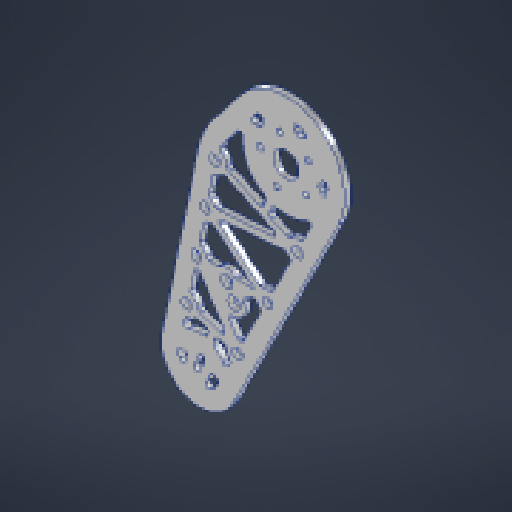
# Autodesk Inventor part: tank_inside_panel
Saved by Autodesk Inventor 2023 (Build 270158000, 158)
## iProperties
Created: 2023-02-28
Part Number: tank_inside_panel
Material: Aluminum 6061
Document SubType Name: Modeling
Designer: ralph
Density: 2.7 g/cm^3
Appearance: Aluminum - Flat
Author: ralph
Autodesk Inventor part; units mm, degrees
(part 1 of 3)
ref_plane "YZ Plane" through (0, 0, 0) normal (1, 0, 0) x (0, 1, 0)
ref_plane "XZ Plane" through (0, 0, 0) normal (0, 1, 0) x (-1, 0, 0)
ref_plane "XY Plane" through (0, 0, 0) normal (0, 0, 1) x (1, 0, 0)
sketch "Sketch1" plane through (0, 0, 0) normal (0, 0, 1) x (1, 0, 0)
  circle A0 centre (-51.8109, -146.0136) radius 3.175 projected
  circle A1 centre (-68.3295, -153.0643) radius 3.175 projected
  line L0 (-87.8947, -227.3231) -> (-92.6287, -239.1078) projected
  arc A2 (-98.521, -236.7409) -> (-92.6287, -239.1078) centre (-95.5749, -237.9244) ccw projected
  line L1 (-98.521, -236.7409) -> (-93.7871, -224.9561) projected
  arc A3 (-87.8947, -227.3231) -> (-93.7871, -224.9561) centre (-90.8409, -226.1396) ccw projected
  circle A4 centre (0, 0) radius 13.4938 projected
  line L2 (-56.4266, -250.7606) -> (56.5866, -28.8133) projected
  arc A5 (56.5866, -28.8133) -> (-50.0843, 39.0361) centre (0, 0) ccw projected
  line L3 (-50.0843, 39.0361) -> (-79.8174, 0.8878) projected
  arc A6 (-79.8174, 0.8878) -> (-94.387, -30.7661) centre (-19.7163, -45.9555) ccw projected
  line L4 (-94.387, -30.7661) -> (-133.6545, -223.8044) projected
  arc A7 (-133.6545, -223.8044) -> (-56.4266, -250.7606) centre (-93.2079, -232.032) ccw projected
  circle A8 centre (-6.7844, 27.1038) radius 3.175 projected
  circle A9 centre (-27.8737, 1.9232) radius 3.175 projected
  circle A10 centre (23.6807, 14.8279) radius 3.175 projected
  circle A11 centre (-10.4425, -25.9152) radius 3.175 projected
  circle A12 centre (21.4199, -17.9397) radius 3.175 projected
  circle A13 centre (12.3652, -76.0452) radius 2.413 projected
  circle A14 centre (-19.9055, -139.4223) radius 2.413 projected
  circle A15 centre (-52.1761, -202.7994) radius 2.413 projected
  line L5 (-60.0746, -215.9418) -> (-61.8773, -219.482) projected
  arc A16 (-67.5567, -219.4404) -> (-61.8773, -219.482) centre (-64.7066, -218.0413) ccw projected
  arc A17 (-109.9237, -202.7115) -> (-105.452, -206.2132) centre (-106.8124, -203.3444) ccw projected
  line L6 (-109.9237, -202.7115) -> (-109.1471, -198.8936) projected
  arc A18 (-106.259, -196.3593) -> (-109.1471, -198.8936) centre (-106.0358, -199.5265) ccw projected
  arc A19 (-106.259, -196.3593) -> (-98.2138, -192.7133) centre (-107.1516, -183.6907) ccw projected
  line L7 (4.4671, -89.1879) -> (-13.923, -125.3043) projected
  arc A20 (-64.7831, -204.3333) -> (-60.7584, -212.1608) centre (-52.1761, -202.7994) ccw projected
  arc A21 (-60.0746, -215.9418) -> (-60.7584, -212.1608) centre (-62.9039, -214.5011) ccw projected
  arc A22 (-92.9229, -119.1359) -> (-91.2544, -122.5971) centre (-89.8116, -119.7688) ccw projected
  line L8 (-92.9229, -119.1359) -> (-88.8946, -99.3326) projected
  arc A23 (-86.0064, -96.7983) -> (-88.8946, -99.3326) centre (-85.7833, -99.9655) ccw projected
  arc A24 (-86.0064, -96.7983) -> (-81.6603, -95.6989) centre (-86.899, -84.1297) ccw projected
  arc A25 (-82.7967, -69.3554) -> (-81.1281, -72.8166) centre (-79.6854, -69.9883) ccw projected
  line L9 (-82.7967, -69.3554) -> (-78.7683, -49.5521) projected
  arc A26 (-75.8802, -47.0178) -> (-78.7683, -49.5521) centre (-75.657, -50.185) ccw projected
  arc A27 (-64.0748, -34.1198) -> (-69.5395, -23.9103) centre (-76.7728, -34.3492) ccw projected
  arc A28 (-70.5556, -19.8503) -> (-69.5395, -23.9103) centre (-67.7312, -21.3006) ccw projected
  arc A29 (-64.7921, -10.8231) -> (-70.5556, -19.8503) centre (-19.7163, -45.9555) ccw projected
  line L10 (-64.7921, -10.8231) -> (-52.5861, 4.8375) projected
  arc A30 (-46.9122, 2.703) -> (-52.5861, 4.8375) centre (-50.0819, 2.8857) ccw projected
  arc A31 (-46.9122, 2.703) -> (-23.4164, -40.7398) centre (0, 0) ccw projected
  arc A32 (26.6735, -45.5766) -> (22.335, -41.3425) centre (23.8442, -44.136) ccw projected
  line L11 (26.6735, -45.5766) -> (18.348, -61.9272) projected
  arc A33 (14.8879, -63.5983) -> (18.348, -61.9272) centre (15.5186, -60.4865) ccw projected
  arc A34 (1.4518, -82.5405) -> (3.7832, -85.4068) centre (12.3652, -76.0452) ccw projected
  arc A35 (4.4671, -89.1879) -> (3.7832, -85.4068) centre (1.6378, -87.7473) ccw projected
  arc A36 (-17.3829, -126.9753) -> (-13.923, -125.3043) centre (-16.7523, -123.8636) ccw projected
  arc A37 (-17.3829, -126.9753) -> (-25.1442, -127.8531) centre (-19.9055, -139.4223) ccw projected
  arc A38 (-63.3886, -164.7638) -> (-63.3439, -164.7448) centre (-68.3295, -153.0643) ccw projected
  line L12 (-63.3439, -164.7448) -> (-46.8252, -157.694) projected
  arc A39 (-46.8252, -157.694) -> (-39.1245, -145.4252) centre (-51.8109, -146.0136) ccw projected
  arc A40 (-35.7266, -142.1112) -> (-39.1245, -145.4252) centre (-35.9529, -145.2781) ccw projected
  line L13 (-35.7266, -142.1112) -> (-34.3965, -142.2063) projected
  arc A41 (-31.6794, -144.183) -> (-34.3965, -142.2063) centre (-34.6229, -145.3732) ccw projected
  arc A42 (-31.6794, -144.183) -> (-28.4876, -148.7838) centre (-19.9055, -139.4223) ccw projected
  arc A43 (-27.8038, -152.5648) -> (-28.4876, -148.7838) centre (-30.6331, -151.1242) ccw projected
  line L14 (-27.8038, -152.5648) -> (-46.1939, -188.6813) projected
  arc A44 (-49.6538, -190.3524) -> (-46.1939, -188.6813) centre (-49.0232, -187.2407) ccw projected
  arc A45 (-49.6538, -190.3524) -> (-50.0192, -190.2839) centre (-52.1761, -202.7994) ccw projected
  arc A46 (-52.1408, -188.8873) -> (-50.0192, -190.2839) centre (-49.48, -187.1551) ccw projected
  line L15 (-52.1408, -188.8873) -> (-64.8141, -169.4209) projected
  arc A47 (-63.3886, -164.7638) -> (-64.8141, -169.4209) centre (-62.1533, -167.6886) ccw projected
  arc A48 (-49.8924, -133.4593) -> (-51.9243, -133.3141) centre (-51.8109, -146.0136) ccw projected
  line L16 (-51.9243, -133.3141) -> (-82.5342, -131.1262) projected
  arc A49 (-85.2514, -129.1495) -> (-82.5342, -131.1262) centre (-82.3079, -127.9593) ccw projected
  arc A50 (-85.2514, -129.1495) -> (-91.2544, -122.5971) centre (-97.0253, -133.9102) ccw projected
  line L17 (-78.3296, -96.1425) -> (-39.1874, -128.4482) projected
  arc A51 (-41.4348, -134.0638) -> (-39.1874, -128.4482) centre (-41.2084, -130.8969) ccw projected
  line L18 (-41.4348, -134.0638) -> (-49.8924, -133.4593) projected
  line L19 (-94.937, -191.9699) -> (-86.0461, -195.0603) projected
  arc A52 (-64.7831, -204.3333) -> (-66.8925, -201.7178) centre (-67.9349, -204.7168) ccw projected
  arc A53 (-94.937, -191.9699) -> (-98.2138, -192.7133) centre (-95.9794, -194.9689) ccw projected
  line L20 (-65.4743, -43.8405) -> (-13.0907, -68.3439) projected
  arc A54 (-14.1782, -74.3844) -> (-13.0907, -68.3439) centre (-14.436, -71.2199) ccw projected
  line L21 (-14.1782, -74.3844) -> (-72.9996, -79.1751) projected
  arc A55 (-75.9857, -77.6344) -> (-72.9996, -79.1751) centre (-73.2574, -76.0105) ccw projected
  arc A56 (-75.9857, -77.6344) -> (-81.1281, -72.8166) centre (-86.899, -84.1297) ccw projected
  arc A57 (-65.4743, -43.8405) -> (-68.8102, -44.243) centre (-66.8195, -46.7164) ccw projected
  line L22 (-28.4749, -127.4095) -> (-71.2037, -92.1436) projected
  arc A58 (-69.4404, -86.5304) -> (-71.2037, -92.1436) centre (-69.1827, -89.6949) ccw projected
  line L23 (-69.4404, -86.5304) -> (-1.5342, -80.9998) projected
  arc A59 (1.4518, -82.5405) -> (-1.5342, -80.9998) centre (-1.2765, -84.1643) ccw projected
  arc A60 (-28.4749, -127.4095) -> (-25.1442, -127.8531) centre (-26.4539, -124.9608) ccw projected
  arc A61 (14.8879, -63.5983) -> (4.4026, -66.1514) centre (12.3652, -76.0452) ccw projected
  arc A62 (1.0667, -66.5539) -> (4.4026, -66.1514) centre (2.4119, -63.6779) ccw projected
  line L24 (1.0667, -66.5539) -> (-16.1603, -58.4956) projected
  arc A63 (-64.0748, -34.1198) -> (-62.2456, -36.9383) centre (-60.9004, -34.0624) ccw projected
  arc A64 (-61.0938, -193.7571) -> (-61.1139, -193.7769) centre (-52.1761, -202.7994) ccw projected
  arc A65 (-64.3907, -194.5202) -> (-61.1139, -193.7769) centre (-63.3483, -191.5212) ccw projected
  line L25 (-64.3907, -194.5202) -> (-92.4352, -184.7723) projected
  arc A66 (-94.5445, -182.1568) -> (-92.4352, -184.7723) centre (-91.3928, -181.7733) ccw projected
  arc A67 (-94.5445, -182.1568) -> (-101.3806, -172.3776) centre (-107.1516, -183.6907) ccw projected
  arc A68 (-103.0492, -168.9165) -> (-101.3806, -172.3776) centre (-99.9379, -169.5493) ccw projected
  line L26 (-103.0492, -168.9165) -> (-99.0208, -149.1131) projected
  arc A69 (-96.1327, -146.5788) -> (-99.0208, -149.1131) centre (-95.9095, -149.746) ccw projected
  arc A70 (-96.1327, -146.5788) -> (-92.3649, -145.7242) centre (-97.0253, -133.9102) ccw projected
  arc A71 (-88.5389, -146.9454) -> (-92.3649, -145.7242) centre (-91.1997, -148.6777) ccw projected
  line L27 (-88.5389, -146.9454) -> (-60.6625, -189.7642) projected
  arc A72 (-61.0938, -193.7571) -> (-60.6625, -189.7642) centre (-63.3233, -191.4965) ccw projected
  arc A73 (-88.6509, -203.8227) -> (-105.452, -206.2132) centre (-93.2079, -232.032) ccw projected
  line L28 (-22.0524, -44.676) -> (-24.5425, -50.8749) projected
  line L29 (-28.8339, -52.5673) -> (-62.2456, -36.9383) projected
  line L30 (-84.1423, -199.2428) -> (-85.1984, -201.8718) projected
  line L31 (-17.7613, -54.4362) -> (-14.9815, -47.5164) projected
  line L32 (-72.8356, -199.6521) -> (-66.8925, -201.7178) projected
  arc A74 (-67.5567, -219.4404) -> (-76.984, -208.5093) centre (-93.2079, -232.032) ccw projected
  arc A75 (-75.8802, -47.0178) -> (-68.8102, -44.243) centre (-76.7728, -34.3492) ccw projected
  line L33 (-78.1275, -204.7122) -> (-76.8242, -201.4676) projected
  arc A76 (-11.2736, -45.6176) -> (22.335, -41.3425) centre (0, 0) ccw projected
  arc A77 (-84.1423, -199.2428) -> (-86.0461, -195.0603) centre (-87.0885, -198.0593) ccw projected
  arc A78 (-88.6509, -203.8227) -> (-85.1984, -201.8718) centre (-88.1445, -200.6883) ccw projected
  arc A79 (-22.0524, -44.676) -> (-23.4164, -40.7398) centre (-24.9986, -43.4925) ccw projected
  arc A80 (-28.8339, -52.5673) -> (-24.5425, -50.8749) centre (-27.4887, -49.6914) ccw projected
  arc A81 (-78.3296, -96.1425) -> (-81.6603, -95.6989) centre (-80.3506, -98.5912) ccw projected
  arc A82 (-72.8356, -199.6521) -> (-76.8242, -201.4676) centre (-73.878, -202.6511) ccw projected
  arc A83 (-78.1275, -204.7122) -> (-76.984, -208.5093) centre (-75.1814, -205.8957) ccw projected
  arc A84 (-11.2736, -45.6176) -> (-14.9815, -47.5164) centre (-12.0354, -48.6999) ccw projected
  arc A85 (-17.7613, -54.4362) -> (-16.1603, -58.4956) centre (-14.8151, -55.6197) ccw projected
  arc A86 (-115.2631, -229.2902) -> (-114.4847, -238.4545) centre (-93.2079, -232.032) ccw projected
  arc A87 (-113.3713, -227.9304) -> (-115.2631, -229.2902) centre (-113.6877, -229.486) ccw projected
  line L34 (-113.3713, -227.9304) -> (-109.5924, -228.6991) projected
  arc A88 (-107.2952, -233.0332) -> (-109.5924, -228.6991) centre (-110.2253, -231.8104) ccw projected
  arc A89 (-107.2952, -233.0332) -> (-108.2711, -237.6145) centre (-95.5749, -237.9244) ccw projected
  arc A90 (-114.4847, -238.4545) -> (-108.2711, -237.6145) centre (-111.4451, -237.537) ccw projected
  arc A91 (-82.9809, -239.5618) -> (-81.2537, -236.3199) centre (-93.2079, -232.032) ccw projected
  arc A92 (-79.039, -235.4413) -> (-81.2537, -236.3199) centre (-79.7594, -236.8559) ccw projected
  line L35 (-79.039, -235.4413) -> (-73.2785, -238.3744) projected
  arc A93 (-72.5842, -240.5094) -> (-73.2785, -238.3744) centre (-73.9989, -239.7891) ccw projected
  line L36 (-72.5842, -240.5094) -> (-73.4026, -242.1166) projected
  arc A94 (-82.2866, -251.3886) -> (-73.4026, -242.1166) centre (-93.2079, -232.032) ccw projected
  arc A95 (-86.1924, -246.4835) -> (-82.2866, -251.3886) centre (-83.8468, -248.6233) ccw projected
  arc A96 (-86.1924, -246.4835) -> (-82.9809, -239.5618) centre (-95.5749, -237.9244) ccw projected
  line L37 (-36.7385, 25.1704) -> (-35.059, 27.3253) projected
  arc A97 (-31.1029, 31.7555) -> (-35.059, 27.3253) centre (0, 0) ccw projected
  arc A98 (-25.7245, 29.1468) -> (-31.1029, 31.7555) centre (-28.8812, 29.4873) ccw projected
  arc A99 (-25.7245, 29.1468) -> (-25.6629, 24.5535) centre (-6.7844, 27.1038) ccw projected
  arc A100 (-28.6757, 20.9563) -> (-25.6629, 24.5535) centre (-28.8093, 24.1285) ccw projected
  arc A101 (-28.6757, 20.9563) -> (-33.3257, 20.1764) centre (-27.8737, 1.9232) ccw projected
  arc A102 (-36.7385, 25.1704) -> (-33.3257, 20.1764) centre (-34.2343, 23.2186) ccw projected
  arc A103 (35.5169, -0.0989) -> (38.7459, 3.1685) centre (23.6807, 14.8279) ccw projected
  arc A104 (44.4304, 1.3195) -> (38.7459, 3.1685) centre (41.2568, 1.2252) ccw projected
  arc A105 (43.8282, -7.409) -> (44.4304, 1.3195) centre (0, 0) ccw projected
  arc A106 (37.9436, -8.4597) -> (43.8282, -7.409) centre (40.6976, -6.8798) ccw projected
  arc A107 (37.9436, -8.4597) -> (35.1939, -4.7799) centre (21.4199, -17.9397) ccw projected
  arc A108 (35.5169, -0.0989) -> (35.1939, -4.7799) centre (37.4896, -2.5866) ccw projected
  arc A109 (11.0693, 33.748) -> (8.9598, 37.8287) centre (-6.7844, 27.1038) ccw projected
  arc A110 (12.4749, 42.6636) -> (8.9598, 37.8287) centre (11.5838, 39.6162) ccw projected
  arc A111 (20.59, 39.3936) -> (12.4749, 42.6636) centre (0, 0) ccw projected
  arc A112 (19.7709, 33.4723) -> (20.59, 39.3936) centre (19.1193, 36.5798) ccw projected
  arc A113 (19.7709, 33.4723) -> (15.4215, 31.9943) centre (23.6807, 14.8279) ccw projected
  arc A114 (11.0693, 33.748) -> (15.4215, 31.9943) centre (14.045, 34.8554) ccw projected
  point P0 (0, 0)
  point P1 (-30.4878, -157.8365)
  point P2 (-86.8989, -84.1298)
  point P3 (-76.7727, -34.3493)
  point P4 (-67.7312, -21.3007)
  point P5 (0, 0)
  constraints: 1 other
extrude "Extrusion1" add sketch "Sketch1" along normal blind 6.35 contours A7 L4 A6 L3 A5 L2 | A8 | A9 | A10 | A11 | A12 | A13 | A14 | A15 | L5 A16 A74 A83 L33 A82 L32 A52 A20 A21 | L6 A18 A19 A53 L19 A77 L30 A78 A73 A17 | L7 A36 A37 A60 L22 A58 L23 A59 A34 A35 | L8 A23 A24 A81 L17 A51 L18 A48 L16 A49 A50 A22 | L9 A26 A75 A57 L20 A54 L21 A55 A56 A25 | A27 A28 A29 L10 A30 A31 A79 L28 A80 L29 A63 | L11 A33 A61 A62 L24 A85 L31 A84 A76 A32 | A38 L12 A39 A40 L13 A41 A42 A43 L14 A44 A45 A46 L15 A47 | A64 A65 L25 A66 A67 A68 L26 A69 A70 A71 L27 A72 | A87 L34 A88 A89 A90 A86 | A91 A92 L35 A93 L36 A94 A95 A96 | L37 A97 A98 A99 A100 A101 A102 | A103 A104 A105 A106 A107 A108 | A109 A110 A111 A112 A113 A114
sketch "Sketch2" plane through (0, 0, 6.35) normal (0, 0, 1) x (1, 0, 0)
  line L0 (-92.6287, -239.1078) -> (-87.8947, -227.3231) projected
  arc A0 (-87.8947, -227.3231) -> (-93.7871, -224.9561) centre (-90.8409, -226.1396) ccw projected
  line L1 (-93.7871, -224.9561) -> (-98.521, -236.7409) projected
  arc A1 (-98.521, -236.7409) -> (-92.6287, -239.1078) centre (-95.5749, -237.9244) ccw projected
  circle A2 centre (0, 0) radius 13.4938 projected
  line L2 (-56.4266, -250.7606) -> (56.5866, -28.8133) projected
  arc A3 (-133.6545, -223.8044) -> (-56.4266, -250.7606) centre (-93.2079, -232.032) ccw projected
  line L3 (-94.387, -30.7661) -> (-133.6545, -223.8044) projected
  arc A4 (-79.8174, 0.8878) -> (-94.387, -30.7661) centre (-19.7163, -45.9555) ccw projected
  line L4 (-50.0843, 39.0361) -> (-79.8174, 0.8878) projected
  arc A5 (56.5866, -28.8133) -> (-50.0843, 39.0361) centre (0, 0) ccw projected
  circle A6 centre (-10.4425, -25.9152) radius 6.731 projected
  circle A7 centre (-6.7844, 27.1038) radius 6.731 projected
  circle A8 centre (-51.8109, -146.0136) radius 6.731 projected
  circle A9 centre (-68.3295, -153.0643) radius 6.731 projected
  circle A10 centre (23.6807, 14.8279) radius 6.731 projected
  circle A11 centre (-27.8737, 1.9232) radius 6.731 projected
  circle A12 centre (21.4199, -17.9397) radius 6.731 projected
  circle A13 centre (-19.9049, -139.4226) radius 5.588 projected
  circle A14 centre (-52.1756, -202.7997) radius 5.588 projected
  circle A15 centre (12.3657, -76.0454) radius 5.588 projected
  arc A16 (-64.7826, -204.3336) -> (-60.7582, -212.1607) centre (-52.1756, -202.7997) ccw projected
  line L5 (18.3479, -61.9273) -> (26.6735, -45.5766) projected
  arc A17 (-94.5445, -182.1568) -> (-101.3806, -172.3776) centre (-107.1516, -183.6907) ccw projected
  arc A18 (-106.259, -196.3593) -> (-109.1471, -198.8936) centre (-106.0358, -199.5265) ccw projected
  line L6 (-109.1471, -198.8936) -> (-109.9237, -202.7115) projected
  arc A19 (-109.9237, -202.7115) -> (-105.452, -206.2132) centre (-106.8124, -203.3444) ccw projected
  arc A20 (-67.5567, -219.4404) -> (-61.8773, -219.482) centre (-64.7066, -218.0413) ccw projected
  line L7 (-61.8773, -219.482) -> (-60.0745, -215.9416) projected
  arc A21 (-60.0745, -215.9416) -> (-60.7582, -212.1607) centre (-62.9039, -214.5009) ccw projected
  arc A22 (-17.3829, -126.9755) -> (-25.1437, -127.8534) centre (-19.9049, -139.4226) ccw projected
  arc A23 (-17.3829, -126.9755) -> (-13.923, -125.3044) centre (-16.7524, -123.8637) ccw projected
  line L8 (-13.923, -125.3044) -> (4.4672, -89.1877) projected
  arc A24 (4.4672, -89.1877) -> (3.7834, -85.4067) centre (1.6379, -87.7471) ccw projected
  arc A25 (14.888, -63.5984) -> (4.4031, -66.1516) centre (12.3657, -76.0454) ccw projected
  arc A26 (14.888, -63.5984) -> (18.3479, -61.9273) centre (15.5186, -60.4867) ccw projected
  arc A27 (26.6735, -45.5766) -> (22.335, -41.3425) centre (23.8442, -44.136) ccw projected
  arc A28 (-11.2736, -45.6176) -> (22.335, -41.3425) centre (0, 0) ccw projected
  arc A29 (-46.9122, 2.703) -> (-52.5861, 4.8375) centre (-50.0819, 2.8857) ccw projected
  line L9 (-52.5861, 4.8375) -> (-64.7921, -10.8231) projected
  arc A30 (-64.7921, -10.8231) -> (-70.5556, -19.8503) centre (-19.7163, -45.9555) ccw projected
  arc A31 (-70.5556, -19.8503) -> (-69.5395, -23.9103) centre (-67.7312, -21.3006) ccw projected
  arc A32 (-64.0748, -34.1198) -> (-69.5395, -23.9103) centre (-76.7728, -34.3492) ccw projected
  arc A33 (-75.8802, -47.0178) -> (-78.7683, -49.5521) centre (-75.657, -50.185) ccw projected
  line L10 (-78.7683, -49.5521) -> (-82.7967, -69.3554) projected
  arc A34 (-82.7967, -69.3554) -> (-81.1281, -72.8166) centre (-79.6854, -69.9883) ccw projected
  arc A35 (-86.0064, -96.7983) -> (-81.6603, -95.6989) centre (-86.899, -84.1297) ccw projected
  arc A36 (-86.0064, -96.7983) -> (-88.8946, -99.3326) centre (-85.7833, -99.9655) ccw projected
  line L11 (-88.8946, -99.3326) -> (-92.9229, -119.1359) projected
  arc A37 (-92.9229, -119.1359) -> (-91.2544, -122.5971) centre (-89.8116, -119.7688) ccw projected
  line L12 (-60.662, -189.7645) -> (-88.5389, -146.9454) projected
  arc A38 (-88.5389, -146.9454) -> (-92.3648, -145.7242) centre (-91.1997, -148.6777) ccw projected
  arc A39 (-96.1327, -146.5788) -> (-92.3648, -145.7242) centre (-97.0253, -133.9102) ccw projected
  arc A40 (-96.1327, -146.5788) -> (-99.0208, -149.1131) centre (-95.9095, -149.746) ccw projected
  line L13 (-99.0208, -149.1131) -> (-103.0492, -168.9165) projected
  arc A41 (-103.0492, -168.9165) -> (-101.3806, -172.3776) centre (-99.9379, -169.5493) ccw projected
  arc A42 (-94.5445, -182.1568) -> (-92.4352, -184.7724) centre (-91.3928, -181.7734) ccw projected
  line L14 (-92.4352, -184.7724) -> (-64.3901, -194.5205) projected
  arc A43 (-64.3901, -194.5205) -> (-61.1133, -193.7771) centre (-63.3477, -191.5215) ccw projected
  arc A44 (-61.0933, -193.7574) -> (-61.1133, -193.7771) centre (-52.1756, -202.7997) ccw projected
  arc A45 (-61.0933, -193.7574) -> (-60.662, -189.7645) centre (-63.3228, -191.4968) ccw projected
  line L15 (-39.187, -128.4483) -> (-78.3296, -96.1425) projected
  arc A46 (-85.2514, -129.1495) -> (-91.2544, -122.5971) centre (-97.0253, -133.9102) ccw projected
  arc A47 (-85.2514, -129.1495) -> (-82.5342, -131.1263) centre (-82.3079, -127.9594) ccw projected
  line L16 (-82.5342, -131.1263) -> (-51.9258, -133.3141) projected
  arc A48 (-49.8908, -133.4595) -> (-51.9258, -133.3141) centre (-51.8109, -146.0136) ccw projected
  line L17 (-49.8908, -133.4595) -> (-41.4344, -134.064) projected
  arc A49 (-41.4344, -134.064) -> (-39.187, -128.4483) centre (-41.208, -130.8971) ccw projected
  line L18 (-34.396, -142.2065) -> (-35.7265, -142.1114) projected
  arc A50 (-35.7265, -142.1114) -> (-39.1245, -145.4254) centre (-35.9529, -145.2783) ccw projected
  arc A51 (-46.8252, -157.694) -> (-39.1245, -145.4254) centre (-51.8109, -146.0136) ccw projected
  line L19 (-46.8252, -157.694) -> (-63.3439, -164.7448) projected
  arc A52 (-63.3884, -164.7637) -> (-63.3439, -164.7448) centre (-68.3295, -153.0643) ccw projected
  arc A53 (-63.3884, -164.7637) -> (-64.8139, -169.4208) centre (-62.1531, -167.6885) ccw projected
  line L20 (-64.8139, -169.4208) -> (-52.1403, -188.8876) projected
  arc A54 (-52.1403, -188.8876) -> (-50.0187, -190.2842) centre (-49.4795, -187.1553) ccw projected
  arc A55 (-49.6537, -190.3526) -> (-50.0187, -190.2842) centre (-52.1756, -202.7997) ccw projected
  arc A56 (-49.6537, -190.3526) -> (-46.194, -188.6815) centre (-49.0233, -187.2408) ccw projected
  line L21 (-46.194, -188.6815) -> (-27.8037, -152.5647) projected
  arc A57 (-27.8037, -152.5647) -> (-28.4874, -148.7837) centre (-30.633, -151.124) ccw projected
  arc A58 (-31.6789, -144.1832) -> (-28.4874, -148.7837) centre (-19.9049, -139.4226) ccw projected
  arc A59 (-31.6789, -144.1832) -> (-34.396, -142.2065) centre (-34.6224, -145.3734) ccw projected
  arc A60 (-106.259, -196.3593) -> (-98.2138, -192.7133) centre (-107.1516, -183.6907) ccw projected
  arc A61 (-64.7826, -204.3336) -> (-66.8919, -201.7181) centre (-67.9343, -204.7171) ccw projected
  line L22 (-86.0461, -195.0603) -> (-94.937, -191.97) projected
  arc A62 (-94.937, -191.97) -> (-98.2138, -192.7133) centre (-95.9794, -194.969) ccw projected
  line L23 (-16.1603, -58.4956) -> (1.0672, -66.5541) projected
  arc A63 (1.0672, -66.5541) -> (4.4031, -66.1516) centre (2.4125, -63.6782) ccw projected
  arc A64 (-64.0748, -34.1198) -> (-62.2456, -36.9383) centre (-60.9004, -34.0624) ccw projected
  arc A65 (-75.8802, -47.0178) -> (-68.8102, -44.243) centre (-76.7728, -34.3492) ccw projected
  arc A66 (-75.9857, -77.6344) -> (-81.1281, -72.8166) centre (-86.899, -84.1297) ccw projected
  arc A67 (-75.9857, -77.6344) -> (-72.9996, -79.1751) centre (-73.2574, -76.0106) ccw projected
  line L24 (-72.9996, -79.1751) -> (-14.1778, -74.3846) projected
  arc A68 (-14.1778, -74.3846) -> (-13.0903, -68.3441) centre (-14.4355, -71.22) ccw projected
  line L25 (-13.0903, -68.3441) -> (-65.4743, -43.8405) projected
  arc A69 (-65.4743, -43.8405) -> (-68.8102, -44.243) centre (-66.8195, -46.7164) ccw projected
  arc A70 (1.4524, -82.5407) -> (3.7834, -85.4067) centre (12.3657, -76.0454) ccw projected
  arc A71 (1.4524, -82.5407) -> (-1.5337, -81) centre (-1.276, -84.1646) ccw projected
  line L26 (-1.5337, -81) -> (-69.4403, -86.5305) projected
  arc A72 (-69.4403, -86.5305) -> (-71.2036, -92.1437) centre (-69.1826, -89.695) ccw projected
  line L27 (-71.2036, -92.1437) -> (-28.4744, -127.4098) projected
  arc A73 (-28.4744, -127.4098) -> (-25.1437, -127.8534) centre (-26.4534, -124.9611) ccw projected
  arc A74 (-67.5567, -219.4404) -> (-76.984, -208.5093) centre (-93.2079, -232.032) ccw projected
  line L28 (-66.8919, -201.7181) -> (-72.8356, -199.6521) projected
  line L29 (-14.9815, -47.5164) -> (-17.7613, -54.4362) projected
  line L30 (-76.8242, -201.4676) -> (-78.1275, -204.7122) projected
  line L31 (-24.5425, -50.8749) -> (-22.0524, -44.676) projected
  arc A75 (-88.6509, -203.8227) -> (-105.452, -206.2132) centre (-93.2079, -232.032) ccw projected
  line L32 (-85.1984, -201.8718) -> (-84.1423, -199.2428) projected
  arc A76 (-46.9122, 2.703) -> (-23.4164, -40.7398) centre (0, 0) ccw projected
  line L33 (-62.2456, -36.9383) -> (-28.8339, -52.5673) projected
  arc A77 (-72.8356, -199.6521) -> (-76.8242, -201.4676) centre (-73.878, -202.6511) ccw projected
  arc A78 (-78.1275, -204.7122) -> (-76.984, -208.5093) centre (-75.1814, -205.8957) ccw projected
  arc A79 (-11.2736, -45.6176) -> (-14.9815, -47.5164) centre (-12.0354, -48.6999) ccw projected
  arc A80 (-17.7613, -54.4362) -> (-16.1603, -58.4956) centre (-14.8151, -55.6197) ccw projected
  arc A81 (-78.3296, -96.1425) -> (-81.6603, -95.6989) centre (-80.3506, -98.5912) ccw projected
  arc A82 (-84.1423, -199.2428) -> (-86.0461, -195.0603) centre (-87.0885, -198.0593) ccw projected
  arc A83 (-88.6509, -203.8227) -> (-85.1984, -201.8718) centre (-88.1445, -200.6883) ccw projected
  arc A84 (-22.0524, -44.676) -> (-23.4164, -40.7398) centre (-24.9986, -43.4925) ccw projected
  arc A85 (-28.8339, -52.5673) -> (-24.5425, -50.8749) centre (-27.4887, -49.6914) ccw projected
  arc A86 (-82.2866, -251.3886) -> (-73.4026, -242.1166) centre (-93.2079, -232.032) ccw projected
  line L34 (-73.4026, -242.1166) -> (-72.5842, -240.5094) projected
  arc A87 (-72.5842, -240.5094) -> (-73.2785, -238.3744) centre (-73.9989, -239.7891) ccw projected
  line L35 (-73.2785, -238.3744) -> (-79.039, -235.4413) projected
  arc A88 (-79.039, -235.4413) -> (-81.2537, -236.3199) centre (-79.7594, -236.8559) ccw projected
  arc A89 (-82.9809, -239.5618) -> (-81.2537, -236.3199) centre (-93.2079, -232.032) ccw projected
  arc A90 (-86.1924, -246.4835) -> (-82.9809, -239.5618) centre (-95.5749, -237.9244) ccw projected
  arc A91 (-86.1924, -246.4835) -> (-82.2866, -251.3886) centre (-83.8468, -248.6233) ccw projected
  arc A92 (-107.2952, -233.0332) -> (-109.5924, -228.6991) centre (-110.2253, -231.8104) ccw projected
  line L36 (-109.5924, -228.6991) -> (-113.3713, -227.9304) projected
  arc A93 (-113.3713, -227.9304) -> (-115.2631, -229.2902) centre (-113.6877, -229.486) ccw projected
  arc A94 (-115.2631, -229.2902) -> (-114.4847, -238.4545) centre (-93.2079, -232.032) ccw projected
  arc A95 (-114.4847, -238.4545) -> (-108.2711, -237.6145) centre (-111.4451, -237.537) ccw projected
  arc A96 (-107.2952, -233.0332) -> (-108.2711, -237.6145) centre (-95.5749, -237.9244) ccw projected
  arc A97 (35.5169, -0.0989) -> (38.7459, 3.1685) centre (23.6807, 14.8279) ccw projected
  arc A98 (35.5169, -0.0989) -> (35.1939, -4.7799) centre (37.4896, -2.5866) ccw projected
  arc A99 (37.9436, -8.4597) -> (35.1939, -4.7799) centre (21.4199, -17.9397) ccw projected
  arc A100 (37.9436, -8.4597) -> (43.8282, -7.409) centre (40.6976, -6.8798) ccw projected
  arc A101 (43.8282, -7.409) -> (44.4304, 1.3195) centre (0, 0) ccw projected
  arc A102 (44.4304, 1.3195) -> (38.7459, 3.1685) centre (41.2568, 1.2252) ccw projected
  arc A103 (11.0693, 33.748) -> (8.9598, 37.8287) centre (-6.7844, 27.1038) ccw projected
  arc A104 (11.0693, 33.748) -> (15.4215, 31.9943) centre (14.045, 34.8554) ccw projected
  arc A105 (19.7709, 33.4723) -> (15.4215, 31.9943) centre (23.6807, 14.8279) ccw projected
  arc A106 (19.7709, 33.4723) -> (20.59, 39.3936) centre (19.1193, 36.5798) ccw projected
  arc A107 (20.59, 39.3936) -> (12.4749, 42.6636) centre (0, 0) ccw projected
  arc A108 (12.4749, 42.6636) -> (8.9598, 37.8287) centre (11.5838, 39.6162) ccw projected
  arc A109 (-31.1029, 31.7555) -> (-35.059, 27.3253) centre (0, 0) ccw projected
  line L37 (-35.059, 27.3253) -> (-36.7385, 25.1704) projected
  arc A110 (-36.7385, 25.1704) -> (-33.3257, 20.1764) centre (-34.2343, 23.2186) ccw projected
  arc A111 (-28.6757, 20.9563) -> (-33.3257, 20.1764) centre (-27.8737, 1.9232) ccw projected
  arc A112 (-28.6757, 20.9563) -> (-25.6629, 24.5535) centre (-28.8093, 24.1285) ccw projected
  arc A113 (-25.7245, 29.1468) -> (-25.6629, 24.5535) centre (-6.7844, 27.1038) ccw projected
  arc A114 (-25.7245, 29.1468) -> (-31.1029, 31.7555) centre (-28.8812, 29.4873) ccw projected
  point P0 (0, 0)
  point P1 (-30.4878, -157.8365)
  point P2 (-86.8983, -84.1302)
  point P3 (0.0004, -0.0002)
extrude "Extrusion2" [suppressed]
sketch "Sketch3" plane through (0, 0, 6.35) normal (0, 0, 1) x (1, 0, 0)
  arc A0 (56.5866, -28.8133) -> (-50.0843, 39.0361) centre (0, 0) ccw projected
  line L0 (-50.0843, 39.0361) -> (-79.8174, 0.8878) projected
  arc A1 (-79.8174, 0.8878) -> (-94.387, -30.7661) centre (-19.7163, -45.9555) ccw projected
  line L1 (-94.387, -30.7661) -> (-133.6545, -223.8044) projected
  arc A2 (-133.6545, -223.8044) -> (-56.4266, -250.7606) centre (-93.2079, -232.032) ccw projected
  line L2 (-56.4266, -250.7606) -> (56.5866, -28.8133) projected
  circle A3 centre (-51.8109, -146.0136) radius 3.175 projected
  circle A4 centre (-68.3295, -153.0643) radius 3.175 projected
  circle A5 centre (0, 0) radius 13.4938 projected
  line L3 (-98.521, -236.7409) -> (-93.7871, -224.9561) projected
  arc A6 (-87.8947, -227.3231) -> (-93.7871, -224.9561) centre (-90.8409, -226.1396) ccw projected
  line L4 (-87.8947, -227.3231) -> (-92.6287, -239.1078) projected
  arc A7 (-98.521, -236.7409) -> (-92.6287, -239.1078) centre (-95.5749, -237.9244) ccw projected
  circle A8 centre (-51.8109, -146.0136) radius 3.175 projected
  line L5 (-51.8109, -146.0136) -> (-63.5956, -141.2796)
  line L6 (-63.5956, -141.2796) -> (-68.3295, -153.0643)
  line L7 (-51.8109, -146.0136) -> (-56.5448, -157.7983)
  line L8 (-56.5448, -157.7983) -> (-68.3295, -153.0643)
  circle A9 centre (-56.5448, -157.7983) radius 3.175
  circle A10 centre (-63.5956, -141.2796) radius 3.175
  point P0 (0, 0)
  dimension "d4" = 6.35
  dimension "d5" = 6.35
  constraints: 8 end point, 4 perpendicular, 2 centre point, 2 coincident
  measures "d4" diameter of A9
  measures "d5" diameter of A10
extrude "Extrusion3" cut sketch "Sketch3" against normal blind 6.35 contours A10 L6 L5 | L5 L6 A10 | A9 L8 L7 | L7 L8 A9
sketch "Sketch4" plane through (0, 0, 6.35) normal (0, 0, 1) x (1, 0, 0)
  circle A0 centre (-56.5448, -157.7983) radius 3.175 projected
  circle A1 centre (-63.5956, -141.2796) radius 3.175 projected
  arc A2 (56.5866, -28.8133) -> (-50.0843, 39.0361) centre (0, 0) ccw projected
  line L0 (-50.0843, 39.0361) -> (-79.8174, 0.8878) projected
  arc A3 (-79.8174, 0.8878) -> (-94.387, -30.7661) centre (-19.7163, -45.9555) ccw projected
  line L1 (-94.387, -30.7661) -> (-133.6545, -223.8044) projected
  arc A4 (-133.6545, -223.8044) -> (-56.4266, -250.7606) centre (-93.2079, -232.032) ccw projected
  line L2 (-56.4266, -250.7606) -> (56.5866, -28.8133) projected
  circle A5 centre (-51.8109, -146.0136) radius 3.175 projected
  circle A6 centre (-68.3295, -153.0643) radius 3.175 projected
  circle A7 centre (0, 0) radius 13.4938 projected
  line L3 (-98.521, -236.7409) -> (-93.7871, -224.9561) projected
  arc A8 (-87.8947, -227.3231) -> (-93.7871, -224.9561) centre (-90.8409, -226.1396) ccw projected
  line L4 (-87.8947, -227.3231) -> (-92.6287, -239.1078) projected
  arc A9 (-98.521, -236.7409) -> (-92.6287, -239.1078) centre (-95.5749, -237.9244) ccw projected
  point P0 (0, 0)
extrude "Extrusion4" add sketch "Sketch4" against normal blind 6.35 contours A5 | A6
chamfer "Chamfer1" distance 3.556 angle 45 2 edges at (-66.7706, -141.2796, 6.35) (-59.7198, -157.7983, 6.35)
sketch "Sketch5" plane through (0, 0, 6.35) normal (0, 0, 1) x (1, 0, 0)
  circle A0 centre (-10.4425, -25.9152) radius 6.731 projected
  circle A1 centre (-6.7844, 27.1038) radius 6.731 projected
  circle A2 centre (-51.8109, -146.0136) radius 6.731 projected
  line L0 (-56.4266, -250.7606) -> (56.5866, -28.8133) projected
  arc A3 (-133.6545, -223.8044) -> (-56.4266, -250.7606) centre (-93.2079, -232.032) ccw projected
  line L1 (-94.387, -30.7661) -> (-133.6545, -223.8044) projected
  arc A4 (-79.8174, 0.8878) -> (-94.387, -30.7661) centre (-19.7163, -45.9555) ccw projected
  line L2 (-50.0843, 39.0361) -> (-79.8174, 0.8878) projected
  arc A5 (56.5866, -28.8133) -> (-50.0843, 39.0361) centre (0, 0) ccw projected
  circle A6 centre (0, 0) radius 13.4938 projected
  line L3 (-92.6287, -239.1078) -> (-87.8947, -227.3231) projected
  arc A7 (-87.8947, -227.3231) -> (-93.7871, -224.9561) centre (-90.8409, -226.1396) ccw projected
  line L4 (-93.7871, -224.9561) -> (-98.521, -236.7409) projected
  arc A8 (-98.521, -236.7409) -> (-92.6287, -239.1078) centre (-95.5749, -237.9244) ccw projected
  circle A9 centre (-68.3295, -153.0643) radius 6.731 projected
  circle A10 centre (23.6807, 14.8279) radius 6.731 projected
  circle A11 centre (-27.8737, 1.9232) radius 6.731 projected
  circle A12 centre (21.4199, -17.9397) radius 6.731 projected
  line L5 (-56.4266, -250.7606) -> (56.5866, -28.8133) projected
  arc A13 (56.5866, -28.8133) -> (-50.0843, 39.0361) centre (0, 0) ccw projected
  line L6 (-50.0843, 39.0361) -> (-79.8174, 0.8878) projected
  arc A14 (-79.8174, 0.8878) -> (-94.387, -30.7661) centre (-19.7163, -45.9555) ccw projected
  line L7 (-94.387, -30.7661) -> (-133.6545, -223.8044) projected
  arc A15 (-133.6545, -223.8044) -> (-56.4266, -250.7606) centre (-93.2079, -232.032) ccw projected
  circle A16 centre (0, 0) radius 13.4938 projected
  line L8 (-87.8947, -227.3231) -> (-92.6287, -239.1078) projected
  arc A17 (-98.521, -236.7409) -> (-92.6287, -239.1078) centre (-95.5749, -237.9244) ccw projected
  line L9 (-98.521, -236.7409) -> (-93.7871, -224.9561) projected
  arc A18 (-87.8947, -227.3231) -> (-93.7871, -224.9561) centre (-90.8409, -226.1396) ccw projected
  circle A19 centre (-68.3295, -153.0643) radius 3.175 projected
  circle A20 centre (-51.8109, -146.0136) radius 3.175 projected
  arc A21 (23.8979, -19.9247) -> (18.9666, -15.9242) centre (21.4446, -17.9092) ccw projected
  arc A22 (18.9666, -15.9242) -> (23.8979, -19.9247) centre (21.4199, -17.9397) ccw projected
  arc A23 (-11.6072, -28.8689) -> (-9.2419, -22.976) centre (-10.4066, -25.9296) ccw projected
  arc A24 (-9.2419, -22.976) -> (-11.6072, -28.8689) centre (-10.4425, -25.9152) ccw projected
  arc A25 (26.3454, 16.5542) -> (20.9946, 13.1351) centre (23.6593, 14.8615) ccw projected
  arc A26 (20.9946, 13.1351) -> (26.3454, 16.5542) centre (23.6807, 14.8279) ccw projected
  arc A27 (-31.0394, 2.1661) -> (-24.7113, 1.6412) centre (-27.877, 1.8842) ccw projected
  arc A28 (-24.7113, 1.6412) -> (-31.0394, 2.1661) centre (-27.8737, 1.9232) ccw projected
  arc A29 (-7.5477, 30.1857) -> (-6.0599, 24.0126) centre (-6.8231, 27.0945) ccw projected
  arc A30 (-6.0599, 24.0126) -> (-7.5477, 30.1857) centre (-6.7844, 27.1038) ccw projected
  circle A31 centre (-19.9055, -139.4223) radius 5.588 projected
  circle A32 centre (-52.1761, -202.7994) radius 5.588 projected
  circle A33 centre (12.3652, -76.0452) radius 5.588 projected
  circle A34 centre (-52.1756, -202.7997) radius 2.413 projected
  circle A35 centre (-19.9049, -139.4226) radius 2.413 projected
  circle A36 centre (12.3657, -76.0454) radius 2.413 projected
  arc A37 (-64.7831, -204.3333) -> (-60.7584, -212.1608) centre (-52.1761, -202.7994) ccw projected
  line L10 (18.348, -61.9272) -> (26.6735, -45.5766) projected
  arc A38 (-94.5445, -182.1568) -> (-101.3806, -172.3776) centre (-107.1516, -183.6907) ccw projected
  arc A39 (-106.259, -196.3593) -> (-109.1471, -198.8936) centre (-106.0358, -199.5265) ccw projected
  line L11 (-109.1471, -198.8936) -> (-109.9237, -202.7115) projected
  arc A40 (-109.9237, -202.7115) -> (-105.452, -206.2132) centre (-106.8124, -203.3444) ccw projected
  arc A41 (-67.5567, -219.4404) -> (-61.8773, -219.482) centre (-64.7066, -218.0413) ccw projected
  line L12 (-61.8773, -219.482) -> (-60.0746, -215.9418) projected
  arc A42 (-60.0746, -215.9418) -> (-60.7584, -212.1608) centre (-62.9039, -214.5011) ccw projected
  arc A43 (-17.3829, -126.9753) -> (-25.1442, -127.8531) centre (-19.9055, -139.4223) ccw projected
  arc A44 (-17.3829, -126.9753) -> (-13.923, -125.3043) centre (-16.7523, -123.8636) ccw projected
  line L13 (-13.923, -125.3043) -> (4.4671, -89.1879) projected
  arc A45 (4.4671, -89.1879) -> (3.7832, -85.4068) centre (1.6378, -87.7473) ccw projected
  arc A46 (14.8879, -63.5983) -> (4.4026, -66.1514) centre (12.3652, -76.0452) ccw projected
  arc A47 (14.8879, -63.5983) -> (18.348, -61.9272) centre (15.5186, -60.4865) ccw projected
  arc A48 (26.6735, -45.5766) -> (22.335, -41.3425) centre (23.8442, -44.136) ccw projected
  arc A49 (-11.2736, -45.6176) -> (22.335, -41.3425) centre (0, 0) ccw projected
  arc A50 (-46.9122, 2.703) -> (-52.5861, 4.8375) centre (-50.0819, 2.8857) ccw projected
  line L14 (-52.5861, 4.8375) -> (-64.7921, -10.8231) projected
  arc A51 (-64.7921, -10.8231) -> (-70.5556, -19.8503) centre (-19.7163, -45.9555) ccw projected
  arc A52 (-70.5556, -19.8503) -> (-69.5395, -23.9103) centre (-67.7312, -21.3006) ccw projected
  arc A53 (-64.0748, -34.1198) -> (-69.5395, -23.9103) centre (-76.7728, -34.3492) ccw projected
  arc A54 (-75.8802, -47.0178) -> (-78.7683, -49.5521) centre (-75.657, -50.185) ccw projected
  line L15 (-78.7683, -49.5521) -> (-82.7967, -69.3554) projected
  arc A55 (-82.7967, -69.3554) -> (-81.1281, -72.8166) centre (-79.6854, -69.9883) ccw projected
  arc A56 (-86.0064, -96.7983) -> (-81.6603, -95.6989) centre (-86.899, -84.1297) ccw projected
  arc A57 (-86.0064, -96.7983) -> (-88.8946, -99.3326) centre (-85.7833, -99.9655) ccw projected
  line L16 (-88.8946, -99.3326) -> (-92.9229, -119.1359) projected
  arc A58 (-92.9229, -119.1359) -> (-91.2544, -122.5971) centre (-89.8116, -119.7688) ccw projected
  line L17 (-60.6625, -189.7642) -> (-88.5389, -146.9454) projected
  arc A59 (-88.5389, -146.9454) -> (-92.3649, -145.7242) centre (-91.1997, -148.6777) ccw projected
  arc A60 (-96.1327, -146.5788) -> (-92.3649, -145.7242) centre (-97.0253, -133.9102) ccw projected
  arc A61 (-96.1327, -146.5788) -> (-99.0208, -149.1131) centre (-95.9095, -149.746) ccw projected
  line L18 (-99.0208, -149.1131) -> (-103.0492, -168.9165) projected
  arc A62 (-103.0492, -168.9165) -> (-101.3806, -172.3776) centre (-99.9379, -169.5493) ccw projected
  arc A63 (-94.5445, -182.1568) -> (-92.4352, -184.7723) centre (-91.3928, -181.7733) ccw projected
  line L19 (-92.4352, -184.7723) -> (-64.3907, -194.5202) projected
  arc A64 (-64.3907, -194.5202) -> (-61.1139, -193.7769) centre (-63.3483, -191.5212) ccw projected
  arc A65 (-61.0938, -193.7571) -> (-61.1139, -193.7769) centre (-52.1761, -202.7994) ccw projected
  arc A66 (-61.0938, -193.7571) -> (-60.6625, -189.7642) centre (-63.3233, -191.4965) ccw projected
  line L20 (-39.1874, -128.4482) -> (-78.3296, -96.1425) projected
  arc A67 (-85.2514, -129.1495) -> (-91.2544, -122.5971) centre (-97.0253, -133.9102) ccw projected
  arc A68 (-85.2514, -129.1495) -> (-82.5342, -131.1262) centre (-82.3079, -127.9593) ccw projected
  line L21 (-82.5342, -131.1262) -> (-51.9243, -133.3141) projected
  arc A69 (-49.8924, -133.4593) -> (-51.9243, -133.3141) centre (-51.8109, -146.0136) ccw projected
  line L22 (-49.8924, -133.4593) -> (-41.4348, -134.0638) projected
  arc A70 (-41.4348, -134.0638) -> (-39.1874, -128.4482) centre (-41.2084, -130.8969) ccw projected
  line L23 (-34.3965, -142.2063) -> (-35.7266, -142.1112) projected
  arc A71 (-35.7266, -142.1112) -> (-39.1245, -145.4252) centre (-35.9529, -145.2781) ccw projected
  arc A72 (-46.8252, -157.694) -> (-39.1245, -145.4252) centre (-51.8109, -146.0136) ccw projected
  line L24 (-46.8252, -157.694) -> (-63.3439, -164.7448) projected
  arc A73 (-63.3886, -164.7638) -> (-63.3439, -164.7448) centre (-68.3295, -153.0643) ccw projected
  arc A74 (-63.3886, -164.7638) -> (-64.8141, -169.4209) centre (-62.1533, -167.6886) ccw projected
  line L25 (-64.8141, -169.4209) -> (-52.1408, -188.8873) projected
  arc A75 (-52.1408, -188.8873) -> (-50.0192, -190.2839) centre (-49.48, -187.1551) ccw projected
  arc A76 (-49.6538, -190.3524) -> (-50.0192, -190.2839) centre (-52.1761, -202.7994) ccw projected
  arc A77 (-49.6538, -190.3524) -> (-46.1939, -188.6813) centre (-49.0232, -187.2407) ccw projected
  line L26 (-46.1939, -188.6813) -> (-27.8038, -152.5648) projected
  arc A78 (-27.8038, -152.5648) -> (-28.4876, -148.7838) centre (-30.6331, -151.1242) ccw projected
  arc A79 (-31.6794, -144.183) -> (-28.4876, -148.7838) centre (-19.9055, -139.4223) ccw projected
  arc A80 (-31.6794, -144.183) -> (-34.3965, -142.2063) centre (-34.6229, -145.3732) ccw projected
  arc A81 (-106.259, -196.3593) -> (-98.2138, -192.7133) centre (-107.1516, -183.6907) ccw projected
  arc A82 (-64.7831, -204.3333) -> (-66.8925, -201.7178) centre (-67.9349, -204.7168) ccw projected
  line L27 (-66.8925, -201.7178) -> (-72.8356, -199.6521) projected
  arc A83 (-94.937, -191.9699) -> (-98.2138, -192.7133) centre (-95.9794, -194.9689) ccw projected
  line L28 (-62.2456, -36.9383) -> (-28.8339, -52.5673) projected
  arc A84 (1.0666, -66.5539) -> (4.4026, -66.1514) centre (2.4119, -63.6779) ccw projected
  arc A85 (-64.0748, -34.1198) -> (-62.2456, -36.9383) centre (-60.9004, -34.0624) ccw projected
  arc A86 (-75.8802, -47.0178) -> (-68.8102, -44.243) centre (-76.7728, -34.3492) ccw projected
  arc A87 (-75.9857, -77.6344) -> (-81.1281, -72.8166) centre (-86.899, -84.1297) ccw projected
  arc A88 (-75.9857, -77.6344) -> (-72.9996, -79.1751) centre (-73.2574, -76.0105) ccw projected
  line L29 (-72.9996, -79.1751) -> (-14.1782, -74.3844) projected
  arc A89 (-14.1782, -74.3844) -> (-13.0907, -68.3439) centre (-14.436, -71.2199) ccw projected
  line L30 (-13.0907, -68.3439) -> (-65.4743, -43.8405) projected
  arc A90 (-65.4743, -43.8405) -> (-68.8102, -44.243) centre (-66.8195, -46.7164) ccw projected
  arc A91 (1.4518, -82.5405) -> (3.7832, -85.4068) centre (12.3652, -76.0452) ccw projected
  arc A92 (1.4518, -82.5405) -> (-1.5342, -80.9998) centre (-1.2765, -84.1643) ccw projected
  line L31 (-1.5342, -80.9998) -> (-69.4404, -86.5304) projected
  arc A93 (-69.4404, -86.5304) -> (-71.2037, -92.1436) centre (-69.1827, -89.6949) ccw projected
  line L32 (-71.2037, -92.1436) -> (-28.4749, -127.4095) projected
  arc A94 (-28.4749, -127.4095) -> (-25.1442, -127.8531) centre (-26.4539, -124.9608) ccw projected
  line L33 (-60.0746, -215.9418) -> (-61.8773, -219.482) projected
  arc A95 (-67.5567, -219.4404) -> (-61.8773, -219.482) centre (-64.7066, -218.0413) ccw projected
  arc A96 (-109.9237, -202.7115) -> (-105.452, -206.2132) centre (-106.8124, -203.3444) ccw projected
  line L34 (-109.9237, -202.7115) -> (-109.1471, -198.8936) projected
  arc A97 (-106.259, -196.3593) -> (-109.1471, -198.8936) centre (-106.0358, -199.5265) ccw projected
  arc A98 (-106.259, -196.3593) -> (-98.2138, -192.7133) centre (-107.1516, -183.6907) ccw projected
  line L35 (4.4671, -89.1879) -> (-13.923, -125.3043) projected
  arc A99 (-64.7826, -204.3336) -> (-60.7582, -212.1607) centre (-52.1756, -202.7997) ccw projected
  arc A100 (-60.0746, -215.9418) -> (-60.7582, -212.1607) centre (-62.9039, -214.5009) ccw projected
  arc A101 (-92.9229, -119.1359) -> (-91.2544, -122.5971) centre (-89.8116, -119.7688) ccw projected
  line L36 (-92.9229, -119.1359) -> (-88.8946, -99.3326) projected
  arc A102 (-86.0064, -96.7983) -> (-88.8946, -99.3326) centre (-85.7833, -99.9655) ccw projected
  arc A103 (-86.0064, -96.7983) -> (-81.6603, -95.6989) centre (-86.899, -84.1297) ccw projected
  arc A104 (-82.7967, -69.3554) -> (-81.1281, -72.8166) centre (-79.6854, -69.9883) ccw projected
  line L37 (-82.7967, -69.3554) -> (-78.7683, -49.5521) projected
  arc A105 (-75.8802, -47.0178) -> (-78.7683, -49.5521) centre (-75.657, -50.185) ccw projected
  arc A106 (-64.0748, -34.1198) -> (-69.5395, -23.9103) centre (-76.7728, -34.3492) ccw projected
  arc A107 (-70.5556, -19.8503) -> (-69.5395, -23.9103) centre (-67.7312, -21.3006) ccw projected
  arc A108 (-64.7921, -10.8231) -> (-70.5556, -19.8503) centre (-19.7163, -45.9555) ccw projected
  line L38 (-64.7921, -10.8231) -> (-52.5861, 4.8375) projected
  arc A109 (-46.9122, 2.703) -> (-52.5861, 4.8375) centre (-50.0819, 2.8857) ccw projected
  arc A110 (-46.9122, 2.703) -> (-23.4164, -40.7398) centre (0, 0) ccw projected
  arc A111 (26.6735, -45.5766) -> (22.335, -41.3425) centre (23.8442, -44.136) ccw projected
  line L39 (26.6735, -45.5766) -> (18.348, -61.9272) projected
  arc A112 (14.888, -63.5984) -> (18.348, -61.9272) centre (15.5186, -60.4867) ccw projected
  arc A113 (1.4524, -82.5407) -> (3.7834, -85.4067) centre (12.3657, -76.0454) ccw projected
  arc A114 (4.4671, -89.1879) -> (3.7834, -85.4067) centre (1.6379, -87.7471) ccw projected
  arc A115 (-17.3829, -126.9755) -> (-13.923, -125.3043) centre (-16.7524, -123.8637) ccw projected
  arc A116 (-17.3829, -126.9755) -> (-25.1437, -127.8534) centre (-19.9049, -139.4226) ccw projected
  arc A117 (-63.3884, -164.7637) -> (-63.3439, -164.7448) centre (-68.3295, -153.0643) ccw projected
  line L40 (-63.3439, -164.7448) -> (-46.8252, -157.694) projected
  arc A118 (-46.8252, -157.694) -> (-39.1245, -145.4254) centre (-51.8109, -146.0136) ccw projected
  arc A119 (-35.7265, -142.1114) -> (-39.1245, -145.4254) centre (-35.9529, -145.2783) ccw projected
  line L41 (-35.7266, -142.1114) -> (-34.3966, -142.2065) projected
  arc A120 (-31.6789, -144.1832) -> (-34.3965, -142.2063) centre (-34.6224, -145.3734) ccw projected
  arc A121 (-31.6789, -144.1832) -> (-28.4874, -148.7837) centre (-19.9049, -139.4226) ccw projected
  arc A122 (-27.8037, -152.5647) -> (-28.4874, -148.7837) centre (-30.633, -151.124) ccw projected
  line L42 (-27.8038, -152.5648) -> (-46.1939, -188.6813) projected
  arc A123 (-49.6537, -190.3526) -> (-46.1939, -188.6813) centre (-49.0233, -187.2408) ccw projected
  arc A124 (-49.6537, -190.3526) -> (-50.0187, -190.2842) centre (-52.1756, -202.7997) ccw projected
  arc A125 (-52.1403, -188.8876) -> (-50.0187, -190.2842) centre (-49.4795, -187.1553) ccw projected
  line L43 (-52.1406, -188.8872) -> (-64.8139, -169.4208) projected
  arc A126 (-63.3884, -164.7637) -> (-64.8141, -169.4209) centre (-62.1531, -167.6885) ccw projected
  arc A127 (-49.8908, -133.4595) -> (-51.9258, -133.3141) centre (-51.8109, -146.0136) ccw projected
  line L44 (-51.9243, -133.3141) -> (-82.5342, -131.1262) projected
  arc A128 (-85.2514, -129.1495) -> (-82.5342, -131.1262) centre (-82.3079, -127.9594) ccw projected
  arc A129 (-85.2514, -129.1495) -> (-91.2544, -122.5971) centre (-97.0253, -133.9102) ccw projected
  line L45 (-78.3296, -96.1425) -> (-39.1874, -128.4481) projected
  arc A130 (-41.4344, -134.064) -> (-39.1874, -128.4482) centre (-41.208, -130.8971) ccw projected
  line L46 (-41.4348, -134.0639) -> (-49.8924, -133.4594) projected
  line L47 (-94.937, -191.97) -> (-86.0461, -195.0603) projected
  arc A131 (-64.7826, -204.3336) -> (-66.8919, -201.7181) centre (-67.9343, -204.7171) ccw projected
  arc A132 (-94.937, -191.97) -> (-98.2138, -192.7133) centre (-95.9794, -194.969) ccw projected
  line L48 (-65.4743, -43.8405) -> (-13.0907, -68.3439) projected
  arc A133 (-14.1778, -74.3846) -> (-13.0907, -68.3439) centre (-14.4355, -71.22) ccw projected
  line L49 (-14.1782, -74.3846) -> (-72.9996, -79.1751) projected
  arc A134 (-75.9857, -77.6344) -> (-72.9996, -79.1751) centre (-73.2574, -76.0106) ccw projected
  arc A135 (-75.9857, -77.6344) -> (-81.1281, -72.8166) centre (-86.899, -84.1297) ccw projected
  arc A136 (-65.4743, -43.8405) -> (-68.8102, -44.243) centre (-66.8195, -46.7164) ccw projected
  line L50 (-28.4748, -127.4094) -> (-71.2037, -92.1436) projected
  arc A137 (-69.4403, -86.5305) -> (-71.2037, -92.1436) centre (-69.1826, -89.695) ccw projected
  line L51 (-69.4404, -86.5305) -> (-1.5342, -81.0001) projected
  arc A138 (1.4524, -82.5407) -> (-1.5342, -80.9998) centre (-1.276, -84.1646) ccw projected
  arc A139 (-28.4749, -127.4095) -> (-25.1437, -127.8534) centre (-26.4534, -124.9611) ccw projected
  arc A140 (14.888, -63.5984) -> (4.4031, -66.1516) centre (12.3657, -76.0454) ccw projected
  arc A141 (1.0672, -66.5541) -> (4.4031, -66.1516) centre (2.4125, -63.6782) ccw projected
  line L52 (1.0672, -66.5541) -> (-16.1603, -58.4956) projected
  arc A142 (-64.0748, -34.1198) -> (-62.2456, -36.9383) centre (-60.9004, -34.0624) ccw projected
  arc A143 (-61.0933, -193.7574) -> (-61.1133, -193.7771) centre (-52.1756, -202.7997) ccw projected
  arc A144 (-64.3901, -194.5205) -> (-61.1133, -193.7771) centre (-63.3477, -191.5215) ccw projected
  line L53 (-64.3907, -194.5202) -> (-92.4352, -184.7723) projected
  arc A145 (-94.5445, -182.1568) -> (-92.4352, -184.7723) centre (-91.3928, -181.7734) ccw projected
  arc A146 (-94.5445, -182.1568) -> (-101.3806, -172.3776) centre (-107.1516, -183.6907) ccw projected
  arc A147 (-103.0492, -168.9165) -> (-101.3806, -172.3776) centre (-99.9379, -169.5493) ccw projected
  line L54 (-103.0492, -168.9165) -> (-99.0208, -149.1131) projected
  arc A148 (-96.1327, -146.5788) -> (-99.0208, -149.1131) centre (-95.9095, -149.746) ccw projected
  arc A149 (-96.1327, -146.5788) -> (-92.3648, -145.7242) centre (-97.0253, -133.9102) ccw projected
  arc A150 (-88.5389, -146.9454) -> (-92.3648, -145.7242) centre (-91.1997, -148.6777) ccw projected
  line L55 (-88.5389, -146.9454) -> (-60.6623, -189.7641) projected
  arc A151 (-61.0933, -193.7574) -> (-60.6625, -189.7642) centre (-63.3228, -191.4968) ccw projected
  arc A152 (-67.5567, -219.4404) -> (-76.984, -208.5093) centre (-93.2079, -232.032) ccw projected
  line L56 (-76.8242, -201.4676) -> (-78.1275, -204.7122) projected
  line L57 (-16.1603, -58.4956) -> (1.0666, -66.5539) projected
  line L58 (-14.9815, -47.5164) -> (-17.7613, -54.4362) projected
  line L59 (-85.1984, -201.8718) -> (-84.1423, -199.2428) projected
  line L60 (-86.0461, -195.0603) -> (-94.937, -191.9699) projected
  arc A153 (-88.6509, -203.8227) -> (-105.452, -206.2132) centre (-93.2079, -232.032) ccw projected
  line L61 (-24.5425, -50.8749) -> (-22.0524, -44.676) projected
  arc A154 (-46.9122, 2.703) -> (-23.4164, -40.7398) centre (0, 0) ccw projected
  arc A155 (-72.8356, -199.6521) -> (-76.8242, -201.4676) centre (-73.878, -202.6511) ccw projected
  arc A156 (-78.1275, -204.7122) -> (-76.984, -208.5093) centre (-75.1814, -205.8957) ccw projected
  arc A157 (-11.2736, -45.6176) -> (-14.9815, -47.5164) centre (-12.0354, -48.6999) ccw projected
  arc A158 (-17.7613, -54.4362) -> (-16.1603, -58.4956) centre (-14.8151, -55.6197) ccw projected
  arc A159 (-78.3296, -96.1425) -> (-81.6603, -95.6989) centre (-80.3506, -98.5912) ccw projected
  arc A160 (-84.1423, -199.2428) -> (-86.0461, -195.0603) centre (-87.0885, -198.0593) ccw projected
  arc A161 (-88.6509, -203.8227) -> (-85.1984, -201.8718) centre (-88.1445, -200.6883) ccw projected
  arc A162 (-22.0524, -44.676) -> (-23.4164, -40.7398) centre (-24.9986, -43.4925) ccw projected
  arc A163 (-28.8339, -52.5673) -> (-24.5425, -50.8749) centre (-27.4887, -49.6914) ccw projected
  arc A164 (-88.6509, -203.8227) -> (-105.452, -206.2132) centre (-93.2079, -232.032) ccw projected
  line L62 (-84.1423, -199.2428) -> (-85.1984, -201.8718) projected
  line L63 (-28.8339, -52.5673) -> (-62.2456, -36.9383) projected
  line L64 (-22.0524, -44.676) -> (-24.5425, -50.8749) projected
  line L65 (-78.1275, -204.7122) -> (-76.8242, -201.4676) projected
  line L66 (-72.8356, -199.6521) -> (-66.8919, -201.7181) projected
  arc A165 (-67.5567, -219.4404) -> (-76.984, -208.5093) centre (-93.2079, -232.032) ccw projected
  arc A166 (-75.8802, -47.0178) -> (-68.8102, -44.243) centre (-76.7728, -34.3492) ccw projected
  line L67 (-17.7613, -54.4362) -> (-14.9815, -47.5164) projected
  arc A167 (-11.2736, -45.6176) -> (22.335, -41.3425) centre (0, 0) ccw projected
  arc A168 (-84.1423, -199.2428) -> (-86.0461, -195.0603) centre (-87.0885, -198.0593) ccw projected
  arc A169 (-88.6509, -203.8227) -> (-85.1984, -201.8718) centre (-88.1445, -200.6883) ccw projected
  arc A170 (-22.0524, -44.676) -> (-23.4164, -40.7398) centre (-24.9986, -43.4925) ccw projected
  arc A171 (-28.8339, -52.5673) -> (-24.5425, -50.8749) centre (-27.4887, -49.6914) ccw projected
  arc A172 (-78.3296, -96.1425) -> (-81.6603, -95.6989) centre (-80.3506, -98.5912) ccw projected
  arc A173 (-72.8356, -199.6521) -> (-76.8242, -201.4676) centre (-73.878, -202.6511) ccw projected
  arc A174 (-78.1275, -204.7122) -> (-76.984, -208.5093) centre (-75.1814, -205.8957) ccw projected
  arc A175 (-11.2736, -45.6176) -> (-14.9815, -47.5164) centre (-12.0354, -48.6999) ccw projected
  arc A176 (-17.7613, -54.4362) -> (-16.1603, -58.4956) centre (-14.8151, -55.6197) ccw projected
  arc A177 (-82.2866, -251.3886) -> (-73.4026, -242.1166) centre (-93.2079, -232.032) ccw projected
  line L68 (-73.4026, -242.1166) -> (-72.5842, -240.5094) projected
  arc A178 (-72.5842, -240.5094) -> (-73.2785, -238.3744) centre (-73.9989, -239.7891) ccw projected
  line L69 (-73.2785, -238.3744) -> (-79.039, -235.4413) projected
  arc A179 (-79.039, -235.4413) -> (-81.2537, -236.3199) centre (-79.7594, -236.8559) ccw projected
  arc A180 (-82.9809, -239.5618) -> (-81.2537, -236.3199) centre (-93.2079, -232.032) ccw projected
  arc A181 (-86.1924, -246.4835) -> (-82.9809, -239.5618) centre (-95.5749, -237.9244) ccw projected
  arc A182 (-86.1924, -246.4835) -> (-82.2866, -251.3886) centre (-83.8468, -248.6233) ccw projected
  arc A183 (-107.2952, -233.0332) -> (-109.5924, -228.6991) centre (-110.2253, -231.8104) ccw projected
  line L70 (-109.5924, -228.6991) -> (-113.3713, -227.9304) projected
  arc A184 (-113.3713, -227.9304) -> (-115.2631, -229.2902) centre (-113.6877, -229.486) ccw projected
  arc A185 (-115.2631, -229.2902) -> (-114.4847, -238.4545) centre (-93.2079, -232.032) ccw projected
  arc A186 (-114.4847, -238.4545) -> (-108.2711, -237.6145) centre (-111.4451, -237.537) ccw projected
  arc A187 (-107.2952, -233.0332) -> (-108.2711, -237.6145) centre (-95.5749, -237.9244) ccw projected
  arc A188 (35.5169, -0.0989) -> (38.7459, 3.1685) centre (23.6807, 14.8279) ccw projected
  arc A189 (35.5169, -0.0989) -> (35.1939, -4.7799) centre (37.4896, -2.5866) ccw projected
  arc A190 (37.9436, -8.4597) -> (35.1939, -4.7799) centre (21.4199, -17.9397) ccw projected
  arc A191 (37.9436, -8.4597) -> (43.8282, -7.409) centre (40.6976, -6.8798) ccw projected
  arc A192 (43.8282, -7.409) -> (44.4304, 1.3195) centre (0, 0) ccw projected
  arc A193 (44.4304, 1.3195) -> (38.7459, 3.1685) centre (41.2568, 1.2252) ccw projected
  arc A194 (11.0693, 33.748) -> (8.9598, 37.8287) centre (-6.7844, 27.1038) ccw projected
  arc A195 (11.0693, 33.748) -> (15.4215, 31.9943) centre (14.045, 34.8554) ccw projected
  arc A196 (19.7709, 33.4723) -> (15.4215, 31.9943) centre (23.6807, 14.8279) ccw projected
  arc A197 (19.7709, 33.4723) -> (20.59, 39.3936) centre (19.1193, 36.5798) ccw projected
  arc A198 (20.59, 39.3936) -> (12.4749, 42.6636) centre (0, 0) ccw projected
  arc A199 (12.4749, 42.6636) -> (8.9598, 37.8287) centre (11.5838, 39.6162) ccw projected
  arc A200 (-31.1029, 31.7555) -> (-35.059, 27.3253) centre (0, 0) ccw projected
  line L71 (-35.059, 27.3253) -> (-36.7385, 25.1704) projected
  arc A201 (-36.7385, 25.1704) -> (-33.3257, 20.1764) centre (-34.2343, 23.2186) ccw projected
  arc A202 (-28.6757, 20.9563) -> (-33.3257, 20.1764) centre (-27.8737, 1.9232) ccw projected
  arc A203 (-28.6757, 20.9563) -> (-25.6629, 24.5535) centre (-28.8093, 24.1285) ccw projected
  arc A204 (-25.7245, 29.1468) -> (-25.6629, 24.5535) centre (-6.7844, 27.1038) ccw projected
  arc A205 (-25.7245, 29.1468) -> (-31.1029, 31.7555) centre (-28.8812, 29.4873) ccw projected
  arc A206 (-115.2631, -229.2902) -> (-114.4847, -238.4545) centre (-93.2079, -232.032) ccw projected
  arc A207 (-113.3713, -227.9304) -> (-115.2631, -229.2902) centre (-113.6877, -229.486) ccw projected
  line L72 (-113.3713, -227.9304) -> (-109.5924, -228.6991) projected
  arc A208 (-107.2952, -233.0332) -> (-109.5924, -228.6991) centre (-110.2253, -231.8104) ccw projected
  arc A209 (-107.2952, -233.0332) -> (-108.2711, -237.6145) centre (-95.5749, -237.9244) ccw projected